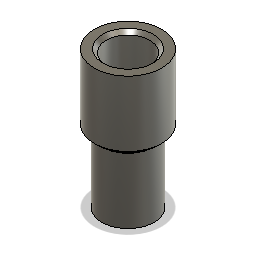
a2m0032_shaft_bushing_v3 (Autodesk Fusion 360 design; units mm, degrees)
Autodesk Fusion 360 part; units mm, degrees
sketch "Sketch1" plane through (0, 0, 0) normal (0, 1, 0) x (1, 0, 0)
  circle A0 centre (0, 0) radius 3.8
  circle A1 centre (0, 0) radius 4.9
  circle A2 centre (0, 0) radius 2.85
  circle A3 centre (0, 0) radius 3.15
  dimension "d1" = 7.6
  dimension "d2" = 9.8
  dimension "d3" = 5.7
  dimension "d4" = 6.3
  constraint coincident A0.centre A1.centre
  constraint concentric A0 A2
  constraint concentric A0 A3
  measures "d1" diameter of A0
  measures "d2" diameter of A1
  measures "d3" diameter of A2
  measures "d4" diameter of A3
extrude "Extrude1" add sketch "Sketch1" against normal blind 10 contours A0 | A3
extrude "Extrude2" add sketch "Sketch1" along normal blind 10 contours A0 | A1
chamfer "Chamfer1" distance 0.5 angle 45 1 edges at (-3.5428, 0, 1.3741)
chamfer "Chamfer2" distance 0.3 angle 45 1 edges at (-2.6571, 0, -1.0306)
chamfer "Chamfer3" distance 0.5 angle 45 2 edges at (-2.6571, -10, 1.0306) (-2.9368, 10, -1.1391)
chamfer "Chamfer4" distance 0.5 angle 45 1 edges at (-4.5684, 0, 1.7719)
